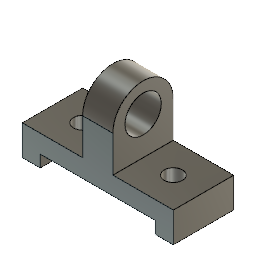
ZAKARIA ABDUL BAQI_UEB0511923_PETROLEUM ENGINEERING_QUIZ 1 v0 (Autodesk Fusion 360 design; units mm, degrees)
Autodesk Fusion 360 part; units mm, degrees
note: some values were not read from the file. Set by a fixed rule: which sketch regions a step uses.
sketch "Sketch1" plane through (0, 0, 0) normal (0, 1, 0) x (1, 0, 0)
  line L0 (10, 0) -> (50, 0)
  line L1 (-50, 0) -> (-50, 20)
  line L2 (-50, 20) -> (-38, 20)
  line L3 (-38, 20) -> (-38, 12)
  line L4 (-38, 12) -> (38, 12)
  line L5 (38, 12) -> (38, 20)
  line L6 (38, 20) -> (50, 20)
  line L7 (50, 20) -> (50, 0)
  line L8 (50, 20) -> (50, 0)
  line L9 (50, 0) -> (10, 0)
  line L10 (50, 0) -> (10, 0)
  line L11 (-10, 0) -> (-50, 0)
  line L12 (-10, 0) -> (-10, -24)
  line L13 (-10, -24) -> (10, -24)
  line L14 (10, -24) -> (10, 0)
  dimension "d1" = 50
  dimension "d2" = 100
  dimension "d3" = 20
  dimension "d4" = 12
  dimension "d5" = 8
  dimension "d6" = 76
  dimension "d7" = 8
  dimension "d8" = 20
  dimension "d9" = 40
  dimension "d13" = 24
  dimension "d14" = 20
  constraint horizontal L0
  constraint parallel L0 L10
  constraint perpendicular L1 L10
  constraint perpendicular L1 L2
  constraint perpendicular L3 L10
  constraint perpendicular L1 L4
  constraint perpendicular L4 L5
  constraint perpendicular L5 L6
  constraint perpendicular L7 L10
  constraint perpendicular L8 L10
  constraint perpendicular L8 L9
  constraint collinear L10 L11
  constraint perpendicular L11 L12
  constraint perpendicular L12 L13
  constraint perpendicular L0 L14
  measures "d1" distance of origin L0.end
  measures "d2" distance of L0.end L1.start
  measures "d3" distance of L1.start L1.end
  measures "d4" distance of L1.end L2.end
  measures "d5" distance of L2.end L3.end
  measures "d6" distance of L3.end L4.end
  measures "d7" distance of L4.end L5.end
  measures "d8" distance of L6.end L0.end
  measures "d9" distance of L0.end L0.start
  measures "d13" distance of L11.start L12.end
  measures "d14" distance of L12.end L13.end
extrude "Extrude1" add sketch "Sketch1" along normal blind 40
sketch "Sketch2" plane through (0, 0, 0) normal (0, 0, 1) x (-1, 0, 0)
  line L0 (-10, 0) -> (-50, 0)
  line L1 (-50, 0) -> (-50, -40)
  line L2 (-50, -40) -> (-10, -40)
  line L3 (-10, -40) -> (-10, 0)
  line L4 (-30, -40) -> (-30, 0)
  circle A0 centre (-30, -20) radius 6
  line L5 (50, 0) -> (30, 0)
  line L6 (30, 0) -> (30, -40)
  circle A1 centre (30, -20) radius 6
  dimension "d17" = 12
  dimension "d18" = 20
  dimension "d19" = 12
  constraint midpoint L2 L4.start
  constraint midpoint L0 L4.end
  constraint midpoint L4 A0.centre
  constraint horizontal L5
  constraint perpendicular L5 L6
  constraint midpoint L6 A1.centre
  measures "d17" diameter of A0
  measures "d18" distance of L5.start L5.end
  measures "d19" diameter of A1
extrude "Extrude2" cut sketch "Sketch2" against normal blind 20 contours L4 A0 | L4 A0
sketch "Sketch3" plane through (0, 0, 0) normal (0, 0, 1) x (-1, 0, 0)
  line L0 (50, 0) -> (10, 0)
  line L1 (10, 0) -> (10, -40)
  line L2 (10, -40) -> (50, -40)
  line L3 (50, -40) -> (50, 0)
  line L4 (50, 0) -> (30, 0)
  line L5 (30, 0) -> (30, -40)
  circle A0 centre (30, -20) radius 6
  dimension "d22" = 12
  constraint coincident L0.start L3.end
  constraint midpoint L0 L4.end
  constraint perpendicular L0 L5
  constraint midpoint L5 A0.centre
  measures "d22" diameter of A0
extrude "Extrude3" cut sketch "Sketch3" against normal blind 20 contours L5 A0 | L5 A0
sketch "Sketch4" plane through (10, 0, 0) normal (1, 0, 0) x (0, 1, 0)
  line L0 (0, 24) -> (0, 0)
  line L1 (0, 0) -> (40, 0)
  line L2 (40, 0) -> (40, 24)
  line L3 (40, 24) -> (0, 24)
  circle A0 centre (20, 24) radius 20
  dimension "d25" = 40
  constraint midpoint L3 A0.centre
  measures "d25" diameter of A0
extrude "Extrude4" add sketch "Sketch4" against normal blind 20 contours L3 A0 picked at (20.4982, 30.648)
sketch "Sketch5" plane through (10, 0, 0) normal (1, 0, 0) x (0, 1, 0)
  line L0 (0, 24) -> (0, 0)
  line L1 (0, 0) -> (40, 0)
  line L2 (40, 0) -> (40, 24)
  arc A0 (40, 24) -> (0, 24) centre (20, 24) ccw
  line L3 (0, 0) -> (0, 25)
  line L4 (0, 25) -> (40, 25)
  circle A1 centre (20, 25) radius 12
  dimension "d28" = 40
  dimension "d29" = 24
  constraint coincident L0.end L1.start
  constraint perpendicular L1 L3
  constraint perpendicular L0 L4
  constraint midpoint L4 A1.centre
  measures "d28" distance of L3.end L4.end
  measures "d29" diameter of A1
extrude "Extrude5" cut sketch "Sketch5" against normal blind 20 contours L4 A1 | L4 A1
sketch "Sketch6" plane through (0, 0, 0) normal (0, -1, 0) x (1, 0, 0)
  line L0 (-10, 24) -> (-10, 0)
  line L1 (-10, 0) -> (-50, 0)
  line L2 (-50, 0) -> (-50, -20)
  line L3 (-50, -20) -> (-38, -20)
  line L4 (-38, -20) -> (-38, -12)
  line L5 (-38, -12) -> (38, -12)
  line L6 (38, -12) -> (38, -20)
  line L7 (38, -20) -> (50, -20)
  line L8 (50, -20) -> (50, 0)
  line L9 (50, 0) -> (10, 0)
  line L10 (10, 0) -> (10, 24)
  line L11 (10, 24) -> (-10, 24)
